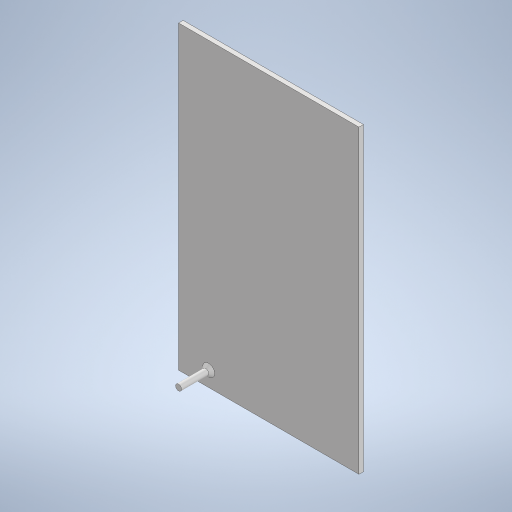
# Autodesk Inventor part: Holder_P1
Saved by Autodesk Inventor 2024 (Build 280153000, 153)
## iProperties
Created: 2023-08-24
Part Number: Holder_P1
Material: Generic
Document SubType Name: Modeling
Designer: l1534
Density: 1 g/cm^3
Appearance: Default
Author: l1534
Autodesk Inventor part; units mm, degrees
ref_plane "YZ Plane" through (0, 0, 0) normal (1, 0, 0) x (0, 1, 0)
ref_plane "XZ Plane" through (0, 0, 0) normal (0, 1, 0) x (-1, 0, 0)
ref_plane "XY Plane" through (0, 0, 0) normal (0, 0, 1) x (1, 0, 0)
sketch "Sketch1" plane through (0, 0, 0) normal (0, 0, 1) x (1, 0, 0)
  line L0 (-78.655, 44.8623) -> (41.345, 44.8623)
  line L1 (41.345, 44.8623) -> (41.345, -155.1377)
  line L2 (41.345, -155.1377) -> (-78.655, -155.1377)
  line L3 (-78.655, -155.1377) -> (-78.655, 44.8623)
  point P0 (0, 0)
  dimension "d1" = 200
  dimension "d2" = 120
  constraints: 8 end point, 2 parallel, 1 horizontal, 1 perpendicular
  measures "d1" distance of L0.end L1.end
  measures "d2" distance of L0.start L0.end
extrude "Extrusion1" add sketch "Sketch1" along normal blind 3
sketch "Sketch2" plane through (0, 0, 3) normal (0, 0, 1) x (1, 0, 0)
  circle A0 centre (-58.655, -145.1377) radius 2
  line L0 (-78.655, -155.1377) -> (41.345, -155.1377) projected
  line L1 (-78.655, 44.8623) -> (-78.655, -155.1377) projected
  point P0 (0, 0)
  dimension "d5" = 4
  dimension "d6" = 10
  dimension "d7" = 20
  constraints: 1 centre point
  measures "d5" diameter of A0
  measures "d6" distance from line of L0 A0.centre
  measures "d7" distance from line of L1 A0.centre
extrude "Extrusion2" add sketch "Sketch2" along normal blind 20
chamfer "Chamfer1" distance 2 angle 45 1 edges at (-60.655, -145.1377, 3)
body "Solid1"
